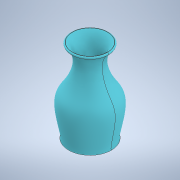
# Autodesk Inventor part: vaseAndFlowers
Saved by Autodesk Inventor 2022 (Build 260153000, 153)
## iProperties
Created: 2023-02-20
Part Number: vaseAndFlowers
Material: Generic
Document SubType Name: Modeling
Designer: mihir
Density: 1 g/cm^3
Appearance: Default
Author: mihir
Autodesk Inventor part; units mm, degrees
ref_plane "YZ Plane" through (0, 0, 0) normal (1, 0, 0) x (0, 1, 0)
ref_plane "XZ Plane" through (0, 0, 0) normal (0, 1, 0) x (-1, 0, 0)
ref_plane "XY Plane" through (0, 0, 0) normal (0, 0, 1) x (1, 0, 0)
sketch "Sketch1" plane through (0, 0, 0) normal (0, 0, 1) x (1, 0, 0)
  line L0 (0, 0) -> (4, 0)
  line L1 (0, 0) -> (0, 15)
  line L2 (0, 0) -> (15, 0) construction
  line L3 (0, 15) -> (4, 15)
  spline S0 degree 4 poles (4, 0) (3.1768, -0.4122) (5.5987, 6.1024) (4.1346, 6.9736) (2.2339, 10.4583) (1.7923, 13.0602) (2.8988, 14.6516) (4, 15) knots 0 0 0 0 0 0.380632 0.534521 0.669654 1 1 1 1 1
  point P0 (4.0252, 1.7661)
  point P1 (4.4569, 6.4638)
  point P2 (3.655, 8.0297)
  point P3 (2.6898, 9.8621)
  point P4 (2.2064, 12.0611)
  point P5 (2.6794, 13.9268)
  point P6 (3.8573, 0)
  dimension "d0" = 4
  dimension "d1" = 15
  dimension "d2" = 90
  dimension "d3" = 4
  constraints: 8 end point, 2 horizontal, 2 perpendicular, 1 vertical, 8 other
  measures "d0" distance of L0.start L0.end
  measures "d1" distance of L0.start L1.end
  measures "d2" angle of L2 L1
  measures "d3" distance of L1.end L3.end
revolve "Revolution1" add sketch "Sketch1" angle 360 about axis through (0, 0, 0) along (0, 1, 0) contours L1 L3 S0 L0
shell "Shell1" thickness 0.4 removed faces 1 at (0.998, 15, 0.8842)
fillet "Fillet1" radius 0.2 1 edges at (-4, 15, 0)
body "Solid1"
